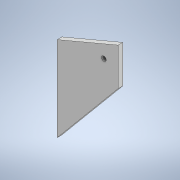
# Autodesk Inventor part: pulley holder
Saved by Autodesk Inventor 2020 (Build 240168000, 168)
## iProperties
Created: 2020-01-24
Part Number: pulley holder
Material: Generic
Document SubType Name: Modeling
Designer: 1jyng
Density: 1 g/cm^3
Appearance: Default
Author: 1jyng
Autodesk Inventor part; units mm, degrees
ref_plane "YZ Plane" through (0, 0, 0) normal (1, 0, 0) x (0, 1, 0)
ref_plane "XZ Plane" through (0, 0, 0) normal (0, 1, 0) x (-1, 0, 0)
ref_plane "XY Plane" through (0, 0, 0) normal (0, 0, 1) x (1, 0, 0)
sketch "Sketch1" plane through (0, 0, 0) normal (0, 0, 1) x (1, 0, 0)
  line L0 (0, 0) -> (0, 114.3)
  line L1 (0, 114.3) -> (81.9127, 148.8473)
  line L2 (81.9127, 148.8473) -> (81.9127, 98.0473)
  line L3 (81.9127, 98.0473) -> (0, 0)
  dimension "d0" = 88.9
  dimension "d1" = 50.8
  dimension "d9" = 114.3
  constraints: 8 end point, 1 parallel, 1 vertical
  measures "d0" distance of L0.end L1.end
  measures "d1" distance of L1.end L2.end
  measures "d9" distance of L0.start L0.end
extrude "Extrusion1" add sketch "Sketch1" along normal blind 6.35
sketch "Sketch2" plane through (0, 0, 6.35) normal (0, 0, 1) x (1, 0, 0)
  circle A0 centre (62.8627, 123.4473) radius 3.175
  line L0 (81.9127, 98.0473) -> (81.9127, 148.8473) projected
  point P0 (0, 0)
  dimension "d4" = 6.35
  dimension "d5" = 19.05
  dimension "d6" = 25.4
  constraints: 1 centre point
  measures "d4" diameter of A0
  measures "d5" distance from line of L0 A0.centre
  measures "d6" vertical distance of L0.end A0.centre
extrude "Extrusion2" cut sketch "Sketch2" against normal blind 6.35
body "Solid1"
